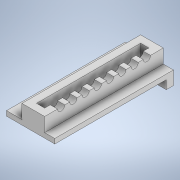
# Autodesk Inventor part: gyro_holder
Saved by Autodesk Inventor 2020 (Build 240168000, 168)
## iProperties
Created: 2019-06-18
Part Number: gyro_holder
Material: Generic
Document SubType Name: Modeling
Designer: erwin
Density: 1 g/cm^3
Appearance: Default
Author: erwin
Autodesk Inventor part; units mm, degrees
ref_plane "YZ Plane" through (0, 0, 0) normal (1, 0, 0) x (0, 1, 0)
ref_plane "XZ Plane" through (0, 0, 0) normal (0, 1, 0) x (-1, 0, 0)
ref_plane "XY Plane" through (0, 0, 0) normal (0, 0, 1) x (1, 0, 0)
sketch "Sketch1" plane through (0, 0, 0) normal (0, 1, 0) x (-1, 0, 0)
  line L0 (0.85, 10.55) -> (-0.85, 10.55)
  line L1 (-0.85, 10.55) -> (-0.85, -10.55)
  line L2 (-0.85, -10.55) -> (0.85, -10.55)
  line L3 (0.85, -10.55) -> (0.85, 10.55)
  line L4 (0.85, 10.55) -> (-0.85, -10.55) construction
  line L5 (-0.85, 10.55) -> (0.85, -10.55) construction
  line L6 (2.35, 12.05) -> (-2.35, 12.05)
  line L7 (-2.35, 12.05) -> (-2.35, -12.05)
  line L8 (-2.35, -12.05) -> (2.35, -12.05)
  line L9 (2.35, -12.05) -> (2.35, 12.05)
  point P0 (0, 0)
  dimension "d0" = 1.7
  dimension "d1" = 21.1
  dimension "d2" = 1.5
  constraints: 20 end point, 4 parallel, 2 midpoint, 2 perpendicular, 1 horizontal, 3 other
  measures "d0" distance of L2.end L1.end
  measures "d1" distance of L1.end L0.end
  measures "d2" distance between parallel lines of L3 L9
extrude "Extrusion1" add sketch "Sketch1" along normal blind 1.5
sketch "Sketch2" plane through (0, 0, 0) normal (0, -1, 0) x (1, 0, 0)
  line L0 (4.95, 12.05) -> (-6.05, 12.05)
  line L1 (-6.05, 12.05) -> (-6.05, -12.05)
  line L2 (-6.05, -12.05) -> (4.95, -12.05)
  line L3 (4.95, -12.05) -> (4.95, 12.05)
  line L4 (-2.35, 12.05) -> (2.35, 12.05) projected
  line L5 (-2.35, -12.05) -> (-2.35, 12.05) projected
  dimension "d5" = 11
  dimension "d6" = 3.7
  constraints: 8 end point, 2 parallel, 1 collinear, 1 horizontal, 1 perpendicular
  measures "d5" distance of L2.end L1.end
  measures "d6" distance between parallel lines of L5 L1
extrude "Extrusion2" add sketch "Sketch2" along normal blind 2.4
sketch "Sketch3" plane through (0, 0, 0) normal (0, 1, 0) x (1, 0, 0)
  line L0 (-2.35, 12.05) -> (-2.35, -12.05) projected
  line L1 (-6.05, 12.05) -> (-2.35, 12.05) projected
  line L2 (-6.05, -12.05) -> (-6.05, 12.05) projected
  line L3 (-2.35, -12.05) -> (-6.05, -12.05) projected
  line L4 (2.35, -12.05) -> (2.35, 12.05) projected
  line L5 (4.95, -12.05) -> (2.35, -12.05) projected
  line L6 (4.95, 12.05) -> (4.95, -12.05) projected
  line L7 (2.35, 12.05) -> (4.95, 12.05) projected
  point P0 (0, 0)
extrude "Extrusion3" cut sketch "Sketch3" against normal blind 1.4
move faces "Move1" translate (0, 0, -1.5) faces at (0.7833, 0.5333, 12.05)
sketch "Sketch4" plane through (0, -2.4, 0) normal (0, -1, 0) x (1, 0, 0)
  line L0 (-0.85, -10.55) -> (0.85, -10.55) projected
  line L1 (-6.05, 10.55) -> (-6.05, -12.05) projected
  line L2 (2.35, -12.05) -> (4.95, -12.05) projected
  line L3 (-6.05, -10.55) -> (4.95, -10.55)
  line L4 (4.95, -10.55) -> (4.95, -12.05)
  line L5 (4.95, -12.05) -> (-6.05, -12.05)
  line L6 (-6.05, -12.05) -> (-6.05, -10.55)
  point P0 (0, 0)
  constraints: 8 end point, 2 parallel, 1 horizontal, 1 perpendicular, 1 point on line
extrude "Extrusion4" add sketch "Sketch4" along normal blind 1.8
move faces "Move2" translate (0, -1.4, 0) faces at (-0.2833, 0, 3.5167)
move faces "Move3" translate (0.5, 0, 0) faces at (-6.05, -1.7333, -4.0167)
move faces "Move4" translate (-0.5, 0, 0) faces at (4.95, -1.7333, -4.0167)
move faces "Move5" translate (0, 0, 1) faces at (-0.65, -2.0667, 10.55)
sketch "Sketch5" plane through (-5.55, -2.4, 11.55) normal (0, 0, 1) x (1, 0, 0)
  line L0 (4.7, 1) -> (4.7, 3.9) projected
  line L1 (3.2, 3.9) -> (4.7, 3.9) projected
  line L2 (3.2, 1) -> (3.2, 3.9) projected
  line L3 (3.2, 1) -> (0, 1) projected
  line L4 (0, 1) -> (0, 0) projected
  line L5 (10, 0) -> (0, 0) projected
  line L6 (10, 1) -> (10, 0) projected
  line L7 (10, 1) -> (7.9, 1) projected
  line L8 (7.9, 1) -> (7.9, 3.9) projected
  line L9 (6.4, 3.9) -> (7.9, 3.9) projected
  line L10 (6.4, 1) -> (6.4, 3.9) projected
  line L11 (6.4, 1) -> (4.7, 1) projected
  line L12 (4.7, 3.9) -> (6.4, 3.9) projected
  line L13 (4.7, 3.9) -> (6.4, 3.9)
  point P0 (5.55, 2.4)
  constraints: 2 end point, 1 collinear
extrude "Extrusion5" add sketch "Sketch5" along normal blind 1
move faces "Move6" translate (0, 0, -0.5) faces at (-0.2833, 0.5333, 11.55)
move faces "Move7" translate (0, 0.5, 0) faces at (-0.85, 0.5333, -3.35) (-0.2833, -1.4, -3.35)
sketch "Sketch6" plane through (2.35, -1.4, -12.05) normal (1, 0, 0) x (0, 0, -1)
  line L0 (-1.5, 2.9) -> (-23.1, 2.9) projected
  circle A0 centre (-3.41, 2.9) radius 0.75
  circle A1 centre (-5.95, 2.9) radius 0.75
  circle A2 centre (-8.49, 2.9) radius 0.75
  circle A3 centre (-11.03, 2.9) radius 0.75
  circle A4 centre (-13.57, 2.9) radius 0.75
  circle A5 centre (-16.11, 2.9) radius 0.75
  circle A6 centre (-18.65, 2.9) radius 0.75
  circle A7 centre (-21.19, 2.9) radius 0.75
  point P0 (-12.05, 1.4)
  dimension "d36" = 1.5
  dimension "d39" = 2.54
  dimension "d44" = 1.91
  dimension "d45" = 1.91
  constraints: 8 centre point, 1 horizontal, 1 point on line, 14 other
  measures "d36" diameter of A0
  measures "d39" distance of A0.centre A1.centre
  measures "d44" distance of L0.start A0.centre
  measures "d45" distance of A7.centre L0.end
extrude "Extrusion6" cut sketch "Sketch6" against normal blind 2
equation "\"d44\" = d45"
body "Solid1"
